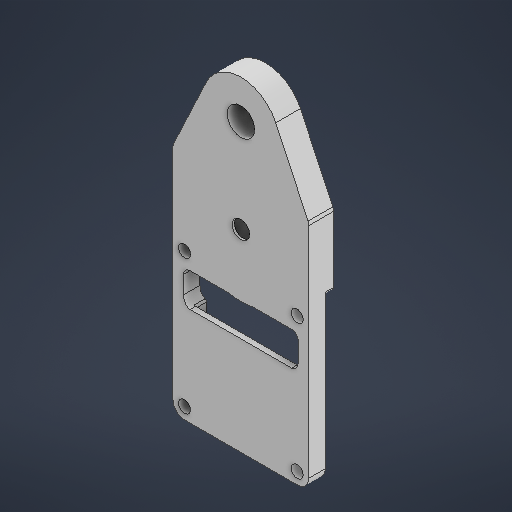
# Autodesk Inventor part: servo_side_plate2
Saved by Autodesk Inventor 2026 (Build 300175000, 175)
## iProperties
Created: 2025-12-05
Part Number: servo_side_plate2
Material: Generic
Document SubType Name: Modeling
Designer: numai
Density: 1 g/cm^3
Appearance: Default
Author: numai
Autodesk Inventor part; units mm, degrees
ref_plane "YZ Plane" through (0, 0, 0) normal (1, 0, 0) x (0, 1, 0)
ref_plane "XZ Plane" through (0, 0, 0) normal (0, 1, 0) x (-1, 0, 0)
ref_plane "XY Plane" through (0, 0, 0) normal (0, 0, 1) x (1, 0, 0)
sketch "スケッチ1" plane through (0, 0, 0) normal (0, 0, 1) x (1, 0, 0)
  circle A0 centre (0, 12.5) radius 5 construction
  line L0 (12.16, 19.2887) -> (12.16, 6.89) construction
  arc A1 (12.16, 19.2887) -> (11.7792, 20.2079) centre (10.86, 19.2887) ccw construction
  line L1 (9.9579, 22.0292) -> (11.7792, 20.2079) construction
  arc A2 (9.9579, 22.0292) -> (9.0387, 22.41) centre (9.0387, 21.11) ccw construction
  line L2 (0.95, 22.41) -> (9.0387, 22.41) construction
  line L3 (0.95, 19.61) -> (0.95, 22.41) construction
  arc A3 (-0.95, 19.61) -> (0.95, 19.61) centre (0, 19.61) ccw construction
  line L4 (-0.95, 22.41) -> (-0.95, 19.61) construction
  line L5 (-9.0387, 22.41) -> (-0.95, 22.41) construction
  arc A4 (-9.0387, 22.41) -> (-9.9579, 22.0292) centre (-9.0387, 21.11) ccw construction
  line L6 (-11.7792, 20.2079) -> (-9.9579, 22.0292) construction
  arc A5 (-11.7792, 20.2079) -> (-12.16, 19.2887) centre (-10.86, 19.2887) ccw construction
  line L7 (-12.16, 6.89) -> (-12.16, 19.2887) construction
  line L8 (-12.16, 6.89) -> (-9.9756, 6.89) construction
  arc A6 (-9.8028, 6.7907) -> (-9.9756, 6.89) centre (-9.9756, 6.69) ccw construction
  arc A7 (-9.8028, 6.7907) -> (-6.5643, 3.2479) centre (0, 12.5) ccw construction
  arc A8 (-6.48, 3.0847) -> (-6.5643, 3.2479) centre (-6.68, 3.0847) ccw construction
  line L9 (-6.48, 3.0847) -> (-6.48, 1.39) construction
  arc A9 (-6.68, 1.19) -> (-6.48, 1.39) centre (-6.68, 1.39) ccw construction
  line L10 (-6.68, 1.19) -> (6.68, 1.19) projected
  arc A10 (6.48, 1.39) -> (6.68, 1.19) centre (6.68, 1.39) ccw construction
  line L11 (6.48, 1.39) -> (6.48, 3.0847) construction
  arc A11 (6.5643, 3.2479) -> (6.48, 3.0847) centre (6.68, 3.0847) ccw construction
  arc A12 (6.5643, 3.2479) -> (9.8028, 6.7907) centre (0, 12.5) ccw construction
  arc A13 (9.9756, 6.89) -> (9.8028, 6.7907) centre (9.9756, 6.69) ccw construction
  line L12 (9.9756, 6.89) -> (12.16, 6.89) construction
  circle A14 centre (0, 29.5) radius 3 projected
  line L13 (-6.3384, 32.4707) -> (-12.2182, 19.9253) projected
  arc A15 (6.3384, 32.4707) -> (-6.3384, 32.4707) centre (0, 29.5) ccw projected
  line L14 (12.2182, 19.9253) -> (6.3384, 32.4707) projected
  arc A16 (12.36, 19.2887) -> (12.2182, 19.9253) centre (10.86, 19.2887) ccw projected
  arc A17 (-12.2182, 19.9253) -> (-12.36, 19.2887) centre (-10.86, 19.2887) ccw projected
  line L15 (12.36, 19.2887) -> (12.36, -20.5) projected
  line L16 (-12.36, -20.5) -> (-12.36, 19.2887) projected
  line L17 (-12.36, 6.89) -> (-9.86, 6.89)
  line L18 (12.36, 6.89) -> (9.86, 6.89)
  arc A18 (-9.86, 6.89) -> (9.86, 6.89) centre (0, 12.5) ccw
  circle A19 centre (0, 12.5) radius 5
  point P0 (0, 0)
  point P1 (-0.8807, 1.19)
  point P2 (0.8807, 1.19)
  dimension "d0" = 10
  constraints: 4 end point, 4 point on line, 3 point on circle, 2 centre point, 2 coincident, 2 horizontal
  measures "d0" diameter of A19
extrude "押し出し1" add sketch "スケッチ1" along normal blind 1.5 contours A18 L17 L16 A17 L13 A15 L14 A16 L15 L18 L10
sketch "スケッチ2" plane through (0, 0, 1.5) normal (0, 0, 1) x (1, 0, 0)
  line L0 (-12.36, 19.2887) -> (-12.36, 6.89) projected
  line L1 (-12.36, 6.89) -> (-9.86, 6.89) projected
  arc A0 (-9.86, 6.89) -> (-0.8807, 1.19) centre (0, 12.5) ccw projected
  line L2 (9.86, 6.89) -> (12.36, 6.89) projected
  line L3 (12.36, 6.89) -> (12.36, 19.2887) projected
  arc A1 (12.36, 19.2887) -> (12.2182, 19.9253) centre (10.86, 19.2887) ccw projected
  line L4 (12.2182, 19.9253) -> (6.3384, 32.4707) projected
  arc A2 (6.3384, 32.4707) -> (-6.3384, 32.4707) centre (0, 29.5) ccw projected
  line L5 (-6.3384, 32.4707) -> (-12.2182, 19.9253) projected
  arc A3 (-12.2182, 19.9253) -> (-12.36, 19.2887) centre (-10.86, 19.2887) ccw projected
  circle A4 centre (0, 29.5) radius 3 projected
  circle A5 centre (0, 12.5) radius 5 projected
  line L6 (9.1914, -4.7213) -> (9.25, -4.7213) projected
  ellipse E0 centre (9.05, -4.9213) end of major axis (9.05, -4.6384) minor radius 0.2 (9.25, -4.9213) -> (9.1914, -4.7213) ccw projected
  line L7 (9.25, -4.9213) -> (9.25, -17.11) projected
  arc A6 (9.05, -17.31) -> (9.25, -17.11) centre (9.05, -17.11) ccw projected
  line L8 (9.05, -17.31) -> (-9.05, -17.31) projected
  arc A7 (-9.25, -17.11) -> (-9.05, -17.31) centre (-9.05, -17.11) ccw projected
  line L9 (-9.25, -17.11) -> (-9.25, -4.9213) projected
  ellipse E1 centre (-9.05, -4.9213) end of major axis (-9.05, -5.2041) minor radius 0.2 (-9.1914, -4.7213) -> (-9.25, -4.9213) ccw projected
  line L10 (-9.25, -4.7213) -> (-9.1914, -4.7213) projected
  ellipse E2 centre (-9.25, -3.0242) end of major axis (-9.25, -4.7213) minor radius 1.2 (-10.45, -3.0242) -> (-9.25, -4.7213) ccw projected
  line L11 (-10.45, 0.19) -> (-10.45, -3.0242) projected
  arc A8 (-9.25, 1.39) -> (-10.45, 0.19) centre (-9.25, 0.19) ccw projected
  line L12 (-6.68, 1.39) -> (-9.25, 1.39) projected
  line L13 (-6.68, 3.0847) -> (-6.68, 1.39) projected
  arc A9 (-9.9756, 6.69) -> (-6.68, 3.0847) centre (0, 12.5) ccw construction
  line L14 (-12.16, 6.69) -> (-9.9756, 6.69) construction
  line L15 (-12.16, -20.5) -> (-12.16, 6.69) construction
  arc A10 (-12.16, -20.5) -> (-10.25, -22.41) centre (-10.25, -20.5) ccw construction
  line L16 (10.25, -22.41) -> (-10.25, -22.41) construction
  arc A11 (10.25, -22.41) -> (12.16, -20.5) centre (10.25, -20.5) ccw construction
  line L17 (12.16, 6.69) -> (12.16, -20.5) construction
  line L18 (9.9756, 6.69) -> (12.16, 6.69) construction
  arc A12 (6.68, 3.0847) -> (9.9756, 6.69) centre (0, 12.5) ccw construction
  line L19 (6.68, 1.39) -> (6.68, 3.0847) projected
  line L20 (9.25, 1.39) -> (6.68, 1.39) projected
  arc A13 (10.45, 0.19) -> (9.25, 1.39) centre (9.25, 0.19) ccw projected
  line L21 (10.45, -3.0242) -> (10.45, 0.19) projected
  ellipse E3 centre (9.25, -3.0242) end of major axis (9.25, -4.7213) minor radius 1.2 (9.25, -4.7213) -> (10.45, -3.0242) ccw projected
  circle A14 centre (10.25, 4) radius 0.7835 construction
  circle A15 centre (10.25, -20.5) radius 0.7835 construction
  circle A16 centre (-10.25, -20.5) radius 0.7835 construction
  circle A17 centre (-10.25, 4) radius 0.7835 construction
  arc A18 (-12.36, -20.5) -> (-10.25, -22.61) centre (-10.25, -20.5) ccw projected
  line L22 (-12.36, 6.69) -> (-12.36, -20.5) projected
  line L23 (-10.25, -22.61) -> (10.25, -22.61) projected
  arc A19 (10.25, -22.61) -> (12.36, -20.5) centre (10.25, -20.5) ccw projected
  line L24 (12.36, -20.5) -> (12.36, 6.69) projected
  line L25 (12.36, 6.69) -> (12.36, 19.2887) projected
  line L26 (-12.36, 19.2887) -> (-12.36, 6.69) projected
  circle A20 centre (-10.25, 4) radius 1.1
  circle A21 centre (-10.25, -20.5) radius 1.1
  circle A22 centre (10.25, -20.5) radius 1.1
  circle A23 centre (10.25, 4) radius 1.1
  line L27 (-6.68, 3.0847) -> (-6.68, 3.3311)
  line L28 (6.68, 3.0847) -> (6.68, 3.3311)
  line L29 (-6.68, 1.39) -> (6.68, 1.39)
  line L30 (-0.8807, 1.19) -> (0.8807, 1.19) projected
  arc A24 (0.8807, 1.19) -> (9.86, 6.89) centre (0, 12.5) ccw projected
  point P0 (0, 0)
  point P1 (-2.2934, 1.39)
  point P2 (2.2934, 1.39)
  dimension "d3" = 2.2
  constraints: 6 end point, 4 centre point, 4 coincident, 3 equal radius, 2 point on circle, 1 horizontal, 1 parallel, 1 vertical, 4 other
  measures "d3" diameter of A20
extrude "押し出し2" add sketch "スケッチ2" along normal blind 2 contours A3 L5 A2 L4 A1 L3 L2 A24 L29 A0 L1 L0 | L1 A0 L27 L13 L12 A8 L11 E2 L10 E1 L9 A7 L8 A6 L7 E0 L6 E3 L21 A13 L20 L19 L28 A24 L2 L25 L24 A19 L23 A18 L22 L26 | A0 L29 L13 L27 | L29 A24 L30 A0 | A24 L28 L19 L29
sketch "スケッチ3" plane through (0, 0, 3.5) normal (0, 0, 1) x (1, 0, 0)
  arc A0 (12.36, 19.2887) -> (12.2182, 19.9253) centre (10.86, 19.2887) ccw projected
  line L0 (12.2182, 19.9253) -> (6.3384, 32.4707) projected
  arc A1 (6.3384, 32.4707) -> (-6.3384, 32.4707) centre (0, 29.5) ccw projected
  line L1 (-6.3384, 32.4707) -> (-12.2182, 19.9253) projected
  arc A2 (-12.2182, 19.9253) -> (-12.36, 19.2887) centre (-10.86, 19.2887) ccw projected
  line L2 (-12.36, 19.2887) -> (-12.36, -20.5) projected
  arc A3 (-12.36, -20.5) -> (-10.25, -22.61) centre (-10.25, -20.5) ccw projected
  line L3 (-10.25, -22.61) -> (10.25, -22.61) projected
  arc A4 (10.25, -22.61) -> (12.36, -20.5) centre (10.25, -20.5) ccw projected
  line L4 (12.36, -20.5) -> (12.36, 19.2887) projected
  arc A5 (-2.2934, 1.39) -> (-0.8807, 1.19) centre (0, 12.5) ccw projected
  line L5 (-0.8807, 1.19) -> (0.8807, 1.19) projected
  arc A6 (0.8807, 1.19) -> (2.2934, 1.39) centre (0, 12.5) ccw projected
  line L6 (2.2934, 1.39) -> (9.25, 1.39) projected
  arc A7 (10.45, 0.19) -> (9.25, 1.39) centre (9.25, 0.19) ccw projected
  line L7 (10.45, 0.19) -> (10.45, -3.0242) projected
  ellipse E0 centre (9.25, -3.0242) end of major axis (9.25, -1.3272) minor radius 1.2 (9.25, -4.7213) -> (10.45, -3.0242) ccw projected
  line L8 (9.25, -4.7213) -> (9.1914, -4.7213) projected
  ellipse E1 centre (9.05, -4.9213) end of major axis (9.05, -5.2041) minor radius 0.2 (9.25, -4.9213) -> (9.1914, -4.7213) ccw projected
  line L9 (9.25, -4.9213) -> (9.25, -17.11) projected
  arc A8 (9.05, -17.31) -> (9.25, -17.11) centre (9.05, -17.11) ccw projected
  line L10 (9.05, -17.31) -> (-9.05, -17.31) projected
  arc A9 (-9.25, -17.11) -> (-9.05, -17.31) centre (-9.05, -17.11) ccw projected
  line L11 (-9.25, -17.11) -> (-9.25, -4.9213) projected
  ellipse E2 centre (-9.05, -4.9213) end of major axis (-9.05, -4.6384) minor radius 0.2 (-9.1914, -4.7213) -> (-9.25, -4.9213) ccw projected
  line L12 (-9.1914, -4.7213) -> (-9.25, -4.7213) projected
  ellipse E3 centre (-9.25, -3.0242) end of major axis (-9.25, -1.3272) minor radius 1.2 (-10.45, -3.0242) -> (-9.25, -4.7213) ccw projected
  line L13 (-10.45, -3.0242) -> (-10.45, 0.19) projected
  arc A10 (-9.25, 1.39) -> (-10.45, 0.19) centre (-9.25, 0.19) ccw projected
  line L14 (-9.25, 1.39) -> (-2.2934, 1.39) projected
  circle A11 centre (0, 29.5) radius 3 projected
  circle A12 centre (0, 12.5) radius 5 projected
  circle A13 centre (-10.25, 4) radius 1.1 projected
  circle A14 centre (-10.25, -20.5) radius 1.1 projected
  circle A15 centre (10.25, -20.5) radius 1.1 projected
  circle A16 centre (10.25, 4) radius 1.1 projected
  line L15 (-9.1914, -4.7213) -> (9.1914, -4.7213)
  point P0 (0, 0)
  constraints: 2 end point, 1 perpendicular, 4 other
extrude "押し出し3" add sketch "スケッチ3" along normal blind 1 contours L4 A4 L3 A3 L2 A2 L1 A1 L0 A0 | L15 E1 L9 A8 L10 A9 L11 E2
sketch "スケッチ4" plane through (0, 0, 4.5) normal (0, 0, 1) x (1, 0, 0)
  circle A0 centre (0, 29.5) radius 3 projected
  circle A1 centre (0, 29.5) radius 2.5
  point P0 (0, 0)
  dimension "d8" = 5
  constraints: 1 centre point, 1 coincident
  measures "d8" diameter of A1
extrude "押し出し4" add sketch "スケッチ4" against normal up to surface (4.5 mm away)
sketch "スケッチ5" plane through (0, 0, 4.5) normal (0, 0, 1) x (1, 0, 0)
  circle A0 centre (0, 12.5) radius 5 projected
  circle A1 centre (0, 12.5) radius 3.05
  point P0 (0, 0)
  dimension "d11" = 6.1
  constraints: 1 centre point, 1 coincident
  measures "d11" diameter of A1
extrude "押し出し5" add sketch "スケッチ5" against normal blind 4
sketch "スケッチ6" plane through (0, 0, 4.5) normal (0, 0, 1) x (1, 0, 0)
  circle A0 centre (0, 12.5) radius 3.05 projected
  circle A1 centre (0, 12.5) radius 1.6
  point P0 (0, 0)
  dimension "d14" = 3.2
  constraints: 1 centre point, 1 coincident
  measures "d14" diameter of A1
extrude "押し出し6" add sketch "スケッチ6" against normal blind 0.4
fillet "フィレット1" radius 0.4 4 edges at (-12.36, 6.89, 0.75) (12.36, 6.89, 0.75) (-9.1914, -4.7213, 2.5) (9.1914, -4.7213, 2.5)
sketch "スケッチ7" plane through (0, 0, 0) normal (0, 0, -1) x (-1, 0, 0)
  circle A0 centre (0, 29.5) radius 2.5 projected
  circle A1 centre (0, 29.5) radius 4.95
  point P0 (0, 0)
  dimension "d18" = 9.9
  constraints: 1 centre point, 1 coincident
  measures "d18" diameter of A1
extrude "押し出し7" add sketch "スケッチ7" along normal blind 1
